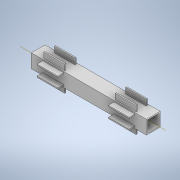
# Autodesk Inventor part: fuselage_tail_interface
Saved by Autodesk Inventor 2021 (Build 250183000, 183)
## iProperties
Created: 2020-11-17
Part Number: fuselage_tail_interface
Material: Generic
Document SubType Name: Modeling
Designer: Paco
Density: 1 g/cm^3
Appearance: Default
Author: Paco
Autodesk Inventor part; units mm, degrees
ref_plane "YZ Plane" through (0, 0, 0) normal (1, 0, 0) x (0, 1, 0)
ref_plane "XZ Plane" through (0, 0, 0) normal (0, 1, 0) x (-1, 0, 0)
sketch "Sketch1" plane through (0, 0, 0) normal (1, 0, 0) x (0, 1, 0)
  line L0 (5.8599, 7.0637) -> (-4.1401, 7.0637)
  line L1 (-4.1401, 7.0637) -> (-4.1401, -2.9363)
  line L2 (-4.1401, -2.9363) -> (5.8599, -2.9363)
  line L3 (5.8599, -2.9363) -> (5.8599, 7.0637)
  line L4 (6.8599, 8.0637) -> (-5.1401, 8.0637)
  line L5 (-5.1401, 8.0637) -> (-5.1401, -3.9363)
  line L6 (-5.1401, -3.9363) -> (6.8599, -3.9363)
  line L7 (6.8599, -3.9363) -> (6.8599, 8.0637)
  point P0 (0, 0)
  dimension "d0" = 10
  dimension "d1" = 10
  dimension "d2" = 12
  dimension "d3" = 12
  dimension "d4" = 1
  dimension "d6" = 1
  constraints: 16 end point, 4 parallel, 2 horizontal, 2 perpendicular
  measures "d0" distance of L0.start L0.end
  measures "d1" distance of L2.end L0.start
  measures "d2" distance of L4.start L4.end
  measures "d3" distance of L4.end L5.end
  measures "d4" distance between parallel lines of L5 L1
  measures "d6" distance between parallel lines of L4 L0
extrude "Extrusion1" add sketch "Sketch1" along normal blind 100
ref_plane "Work Plane1" through (0, -5.1401, 2.0637) normal (0, 0, 1) x (1, 0, 0)
ref_plane "Work Plane2" through (0, 0.8599, 8.0637) normal (0, 1, 0) x (1, 0, 0)
ref_plane "Work Plane3" through (0, -5.1401, 6.0637) normal (0, 0, 1) x (1, 0, 0)
sketch "Sketch3" plane through (0, -5.1401, 6.0637) normal (0, 0, 1) x (1, 0, 0)
  line L0 (0, 12) -> (100, 12) projected
  line L1 (10, 12) -> (28, 12)
  line L2 (28, 12) -> (28, 17)
  line L3 (28, 17) -> (10, 17)
  line L4 (10, 17) -> (10, 12)
  line L5 (72, 12) -> (90, 12)
  line L6 (90, 12) -> (90, 17)
  line L7 (90, 17) -> (72, 17)
  line L8 (72, 17) -> (72, 12)
  line L9 (100, 12) -> (100, 0) projected
  line L10 (0, 12) -> (0, 0) projected
  line L11 (50, 21.2815) -> (50, -16.5994)
  point P0 (0, 5.1401)
  dimension "d10" = 18
  dimension "d11" = 18
  dimension "d12" = 100
  dimension "d13" = 50
  dimension "d15" = 10
  dimension "d16" = 10
  dimension "d17" = 5
  constraints: 18 end point, 4 parallel, 3 point on line, 2 horizontal, 2 perpendicular, 1 vertical
  measures "d10" distance of L2.end L3.end
  measures "d11" distance of L6.end L7.end
  measures "d12" distance between parallel lines of L9 L10
  measures "d13" distance between parallel lines of L9 L11
  measures "d15" distance between parallel lines of L10 L4
  measures "d16" distance between parallel lines of L9 L6
  measures "d17" distance of L7.end L5.start
extrude "Extrusion2" add sketch "Sketch3" along normal blind 1
mirror "Mirror1" about plane through (0, -5.1401, 2.0637) normal (0, 0, 1) of "Extrusion2"
mirror "Mirror2" about plane through (0, 0.8599, 8.0637) normal (0, 1, 0) of "Extrusion2", "Mirror1"
pattern_circular "Circular Pattern1" count 2 over 270 about axis through (0, 0.8599, 2.0637) along (-1, 0, 0) of "Extrusion2", "Mirror1"
equation "\"d1\" = d0"
equation "\"d3\" = d2"
equation "\"d11\" = d10"
equation "\"d13\" = 0.5 * d12"
equation "\"d15\" = 0.1 * d12"
equation "\"d16\" = d15"
body "Solid1"
